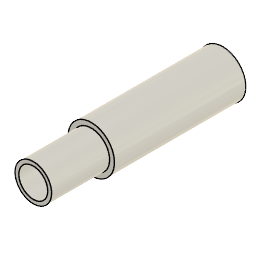
Spit-Bar v10 (Autodesk Fusion 360 design; units mm, degrees)
Autodesk Fusion 360 part; units mm, degrees
sketch "Sketch1" plane through (0, 0, 0) normal (0, 1, 0) x (1, 0, 0)
  circle A0 centre (0, 0) radius 12
  circle A1 centre (0, 0) radius 7.5
  circle A2 centre (0, 0) radius 9.5
  constraint coincident A0.centre A1.centre
  constraint concentric A0 A2
extrude "Extrude1" add sketch "Sketch1" along normal blind 45 contours A0 | A2
extrude "Extrude2" add sketch "Sketch1" against normal blind 25 contours A2
extrude "Extrude3" add sketch "Sketch1" against normal blind 11 contours A0
extrude "Extrude4" add 1 faces at (8.77, -25, 0.8446) along direction (0, -1, 0) blind 16
extrude "Extrude5" add 1 faces at (11.0866, -11, 1.0681) along direction (0, -1, 0) blind 14
extrude "Extrude6" add 1 faces at (8.77, -41, 0.8446) along direction (0, -1, 0) blind 14
extrude "Extrude8" cut 1 faces at (10.4274, 45, 0.9688) along direction (0, -1, 0) blind 2
extrude "Extrude7" [suppressed]
